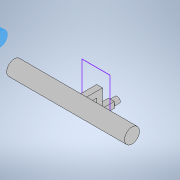
# Autodesk Inventor part: ONLY_Inventor_inv1
Saved by Autodesk Inventor 2020.3 (Build 243373000, 373)
## iProperties
Created: 2021-03-02
Part Number: ONLY_Inventor_inv1
Material: Generisch
Document SubType Name: Modeling
Designer: Stefan
Density: 1 g/cm^3
Appearance: Vorgabe
Author: Stefan
Autodesk Inventor part; units mm, degrees
ref_plane "YZ Plane" through (0, 0, 0) normal (1, 0, 0) x (0, 1, 0)
ref_plane "XZ Plane" through (0, 0, 0) normal (0, 1, 0) x (-1, 0, 0)
ref_plane "XY Plane" through (0, 0, 0) normal (0, 0, 1) x (1, 0, 0)
sketch "Skizze1" plane through (0, 0, 0) normal (0, 0, 1) x (1, 0, 0)
  circle A0 centre (0, 0) radius 5
  dimension "d0" = 10
  constraints: 1 centre point, 1 coincident
  measures "d0" diameter of A0
extrude "Extrusion1" add sketch "Skizze1" along normal blind 10
sketch "Skizze2" plane through (0, 0, 10) normal (0, 0, 1) x (1, 0, 0)
  line L0 (-5, 5) -> (5, 5)
  line L1 (5, 5) -> (5, -5)
  line L2 (5, -5) -> (-5, -5)
  line L3 (-5, -5) -> (-5, 5)
  circle A0 centre (0, 0) radius 5 projected
  dimension "d3" = 10
  dimension "d4" = 10
  constraints: 8 end point, 2 parallel, 2 tangent, 1 horizontal, 1 perpendicular
  measures "d3" distance of L1.end L2.end
  measures "d4" distance of L0.end L1.end
extrude "Extrusion2" add sketch "Skizze2" along normal blind 30
sketch "Skizze3" plane through (0, 5, 10) normal (0, 1, 0) x (1, 0, 0)
  line L0 (-5, -30) -> (5, -30) projected
  line L1 (5, -30) -> (-5, -30)
  line L2 (-5, -30) -> (-5, -20)
  line L3 (-5, -20) -> (5, -20)
  line L4 (5, -20) -> (5, -30)
  point P0 (0, 10)
  dimension "d7" = 10
  dimension "d8" = 10
  constraints: 8 end point, 2 parallel, 1 horizontal, 1 perpendicular
  measures "d7" distance of L2.end L3.end
  measures "d8" distance of L1.end L2.end
extrude "Extrusion3" add sketch "Skizze3" along normal blind 30
sketch "Skizze5" plane through (0, 0, 40) normal (0, 0, 1) x (1, 0, 0)
  line L0 (-5, -5) -> (-5, 35) projected
  line L1 (-5, 35) -> (5, 35)
  line L2 (5, 35) -> (5, 25)
  line L3 (5, 25) -> (-5, 25)
  line L4 (-5, 25) -> (-5, 35)
  point P0 (0, 0)
  dimension "d11" = 10
  dimension "d12" = 10
  constraints: 8 end point, 2 parallel, 1 horizontal, 1 perpendicular
  measures "d11" distance of L2.end L3.end
  measures "d12" distance of L1.end L2.end
extrude "Extrusion4" add sketch "Skizze5" along normal blind 30
sketch "Skizze6" plane through (-5, 0, 10) normal (-1, 0, 0) x (0, 0, 1)
  line L0 (60, 25) -> (60, 35) projected
  circle A0 centre (60, 30) radius 12.65
  point P0 (-10, 0)
  dimension "d15" = 25.3
  constraints: 1 centre point, 1 midpoint
  measures "d15" diameter of A0
extrude "Extrusion5" add sketch "Skizze6" along normal mid plane 200
sketch "Skizze7" plane through (0, 0, 40) normal (0, 0, 1) x (1, 0, 0)
  line L0 (-22.05, -0.6125) -> (22.05, -0.6125)
  line L1 (22.05, -0.6125) -> (22.05, 64.7208)
  line L2 (22.05, 64.7208) -> (-22.05, 64.7208)
  line L3 (-22.05, 64.7208) -> (-22.05, -0.6125)
  line L4 (-5, 5) -> (-5, 35) projected
  point P0 (0, 0)
  dimension "d18" = 44.1
  dimension "d19" = 17.05
  constraints: 8 end point, 2 parallel, 1 horizontal, 1 perpendicular
  measures "d18" distance of L1.end L2.end
  measures "d19" distance between parallel lines of L3 L4
extrude "Extrusion6" add sketch "Skizze7" along normal blind 50
